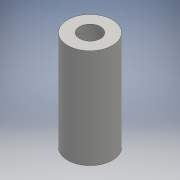
# Autodesk Inventor part: PcbSpacer4x20mm
Saved by Autodesk Inventor 2016 (Build 200138000, 138)
## iProperties
Created: 2026-04-02
Part Number: PcbSpacer4x20mm
Material: Generic
Document SubType Name: Modeling
Designer: Steve
Density: 1 g/cm^3
Appearance: Default
Author: Steve
Autodesk Inventor part; units mm, degrees
ref_plane "YZ Plane" through (0, 0, 0) normal (1, 0, 0) x (0, 1, 0)
ref_plane "XZ Plane" through (0, 0, 0) normal (0, 1, 0) x (-1, 0, 0)
ref_plane "XY Plane" through (0, 0, 0) normal (0, 0, 1) x (1, 0, 0)
sketch "Sketch1" plane through (0, 0, 0) normal (0, 0, 1) x (1, 0, 0)
  circle A0 centre (0, 0) radius 4.5
  circle A1 centre (0, 0) radius 2.1
  dimension "d0" = 9
  dimension "d1" = 4.2
  constraints: 2 centre point, 2 coincident
  measures "d0" diameter of A0
  measures "d1" diameter of A1
extrude "Extrusion1" add sketch "Sketch1" along normal blind 20
body "Solid1"
